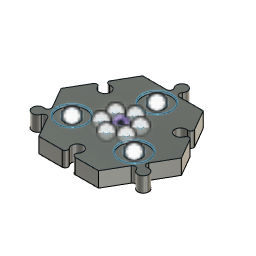
Fushion puzzle 1.0 CAD (Autodesk Fusion 360 design; units mm, degrees)
Autodesk Fusion 360 part; units mm, degrees
note: some values were not read from the file. Set by a fixed rule: which face or edge a step refers to.
sketch "Sketch1" plane through (0, 0, 0) normal (0, 0, 1) x (1, 0, 0)
  line L0 (42, 0) -> (21, 36.3731)
  line L1 (21, 36.3731) -> (-21, 36.3731)
  line L2 (-21, 36.3731) -> (-42, 0)
  line L3 (-42, 0) -> (-21, -36.3731)
  line L4 (-21, -36.3731) -> (21, -36.3731)
  line L5 (21, -36.3731) -> (42, 0)
  circle A0 centre (0, 42.3731) radius 4
  line L6 (0, 41) -> (0, 36.3731)
  arc A1 (2.9814, 39.7064) -> (4.4721, 36.3731) centre (4.4721, 38.3731) ccw
  arc A2 (-4.4721, 36.3731) -> (-2.9814, 39.7064) centre (-4.4721, 38.3731) ccw
  circle A3 centre (-36.6962, -21.1865) radius 4
  arc A4 (-29.2639, -22.0595) -> (-32.896, -22.4352) centre (-30.996, -23.0595) ccw
  arc A5 (-35.8775, -17.2712) -> (-33.7361, -14.3136) centre (-35.4681, -15.3136) ccw
  circle A6 centre (36.6962, -21.1865) radius 4
  arc A7 (33.7361, -14.3136) -> (35.8775, -17.2712) centre (35.4681, -15.3136) ccw
  arc A8 (32.896, -22.4352) -> (29.2639, -22.0595) centre (30.996, -23.0595) ccw
  circle A9 centre (-26.3038, 15.1865) radius 4
  arc A10 (-29.2639, 22.0595) -> (-27.1225, 19.1019) centre (-27.5319, 21.0595) ccw
  arc A11 (-30.104, 13.9379) -> (-33.7361, 14.3136) centre (-32.004, 13.3136) ccw
  circle A12 centre (0, -30.3731) radius 4
  arc A13 (-4.4721, -36.3731) -> (-2.9814, -33.0397) centre (-4.4721, -34.3731) ccw
  arc A14 (2.9814, -33.0397) -> (4.4721, -36.3731) centre (4.4721, -34.3731) ccw
  circle A15 centre (26.3038, 15.1865) radius 4
  arc A16 (33.7361, 14.3136) -> (30.104, 13.9379) centre (32.004, 13.3136) ccw
  arc A17 (27.1225, 19.1019) -> (29.2639, 22.0595) centre (27.5319, 21.0595) ccw
  dimension "d1" = 42
  dimension "d2" = 8
  dimension "d3" = 6
  dimension "d4" = 4
  dimension "d6" = 360
  dimension "d10" = 360
  constraint tangent A0 A2
  constraint tangent L1 A2
  constraint vertical L6
  constraint symmetric L6 A1 A2
  constraint coincident L1 L6.end
  constraint coincident L1 A1.end
  constraint coincident A0 A1.start
  constraint coincident A0 A2.end
  constraint coincident L1 A2.start
  measures "d1" distance of L0.end L1.end
  measures "d2" diameter of A0
  measures "d3" distance of L1 A0.centre
  measures "d4" diameter of A2
extrude "Extrude1" add sketch "Sketch1" along normal blind 10.5 contours L0 L1 L2 L3 L4 L5 A9 A10 A11 A12 A13 A14 A15 A16 A17 | L5 A6 A7 A8 | A6 | L1 A0 L6 A1 | L1 A0 L6 A2 | A0 | L3 A3 A4 A5 | A3
move_face "OffsetFaces1" offset -0.2 9 faces at (39.0509, -24.42, 7) (29.3138, -21.9777, 7) (-37.9917, -24.9709, 7) (-30.5353, -21.1133, 7) (34.8369, -17.2113, 7) (3.9953, 42.1785, 7) (2.513, 38.7754, 7) (-34.8369, -17.2113, 7) (-2.513, 38.7754, 7)
sketch "Sketch2" plane through (0, 0, 10.5) normal (0, 0, 1) x (-1, 0, 0)
  line L0 (-33.5629, 14.2136) -> (-41.8845, -0.2)
  line L1 (-41.8845, -0.2) -> (-33.7361, -14.3136)
  arc A0 (-33.7361, -14.3136) -> (-30.104, -13.9379) centre (-32.004, -13.3136) ccw
  arc A1 (-27.1225, -19.1019) -> (-30.104, -13.9379) centre (-26.3038, -15.1865) ccw
  arc A2 (-27.1225, -19.1019) -> (-29.2639, -22.0595) centre (-27.5319, -21.0595) ccw
  line L2 (-29.2639, -22.0595) -> (-21.1155, -36.1731)
  line L3 (-21.1155, -36.1731) -> (-4.4721, -36.1731)
  arc A3 (-2.8324, -39.8397) -> (-4.4721, -36.1731) centre (-4.4721, -38.3731) ccw
  arc A4 (-2.8324, -39.8397) -> (2.8324, -39.8397) centre (0, -42.3731) ccw
  arc A5 (4.4721, -36.1731) -> (2.8324, -39.8397) centre (4.4721, -38.3731) ccw
  line L4 (4.4721, -36.1731) -> (21.1155, -36.1731)
  line L5 (21.1155, -36.1731) -> (29.2639, -22.0595)
  arc A6 (29.2639, -22.0595) -> (27.1225, -19.1019) centre (27.5319, -21.0595) ccw
  arc A7 (30.104, -13.9379) -> (27.1225, -19.1019) centre (26.3038, -15.1865) ccw
  arc A8 (30.104, -13.9379) -> (33.7361, -14.3136) centre (32.004, -13.3136) ccw
  line L6 (33.7361, -14.3136) -> (41.8845, -0.2)
  line L7 (41.8845, -0.2) -> (33.5629, 14.2136)
  arc A9 (35.9184, 17.467) -> (33.5629, 14.2136) centre (35.4681, 15.3136) ccw
  arc A10 (35.9184, 17.467) -> (33.086, 22.3728) centre (36.6962, 21.1865) ccw
  arc A11 (29.0907, 21.9595) -> (33.086, 22.3728) centre (30.996, 23.0595) ccw
  line L8 (29.0907, 21.9595) -> (20.7691, 36.3731)
  line L9 (20.7691, 36.3731) -> (4.4721, 36.3731)
  arc A12 (4.4721, 36.3731) -> (2.9814, 33.0397) centre (4.4721, 34.3731) ccw
  arc A13 (-2.9814, 33.0397) -> (2.9814, 33.0397) centre (0, 30.3731) ccw
  arc A14 (-2.9814, 33.0397) -> (-4.4721, 36.3731) centre (-4.4721, 34.3731) ccw
  line L10 (-4.4721, 36.3731) -> (-20.7691, 36.3731)
  line L11 (-20.7691, 36.3731) -> (-29.0907, 21.9595)
  arc A15 (-33.086, 22.3728) -> (-29.0907, 21.9595) centre (-30.996, 23.0595) ccw
  arc A16 (-33.086, 22.3728) -> (-35.9184, 17.467) centre (-36.6962, 21.1865) ccw
  arc A17 (-33.5629, 14.2136) -> (-35.9184, 17.467) centre (-35.4681, 15.3136) ccw
  circle A18 centre (0, -25) radius 10
  circle A19 centre (0, -25) radius 5
  circle A20 centre (0, -10) radius 1.75
  circle A21 centre (21.6506, 12.5) radius 5
  circle A22 centre (21.6506, 12.5) radius 10
  circle A23 centre (-21.6506, 12.5) radius 5
  circle A24 centre (-21.6506, 12.5) radius 10
  circle A25 centre (8.6603, -5) radius 1.75
  circle A26 centre (8.6603, 5) radius 1.75
  circle A27 centre (0, 10) radius 1.75
  circle A28 centre (-8.6603, 5) radius 1.75
  circle A29 centre (-8.6603, -5) radius 1.75
  dimension "d14" = 10
  dimension "d15" = 20
  dimension "d16" = 3.5
  dimension "d18" = 360
  dimension "d20" = 360
  constraint concentric A18 A19
  measures "d14" diameter of A19
  measures "d15" diameter of A18
  measures "d16" diameter of A20
extrude "Extrude2" cut sketch "Sketch2" against normal blind 1.5 contours A18 | A22 | A24
extrude "Extrude3" cut 3 faces at (-2.3344, 25.4913, 10.5) (-21.8157, -11.3785, 10.5) (21.4856, -11.3785, 10.5) along direction (0, 0, -1) blind 6
extrude "Extrude4" cut sketch "Sketch2" against normal blind 5 contours A20 | A25 | A26 | A27 | A28 | A29
